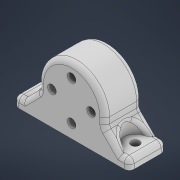
# Autodesk Inventor part: 15mm Hex Hub
Saved by Autodesk Inventor 2022 (Build 260153000, 153)
## iProperties
Created: 2021-11-10
Part Number: 15mm Hex Hub
Material: Generic
Document SubType Name: Modeling
Designer: izack
Density: 1 g/cm^3
Appearance: Default
Author: izack
## iProperties of the stored document 15mm Hex Hub_3DPrint.ipt
Part Number: 15mm Hex Hub_3DPrint
Material: Generic
Document SubType Name: Modeling
Designer: izack
Appearance: Default
Author: izack
Autodesk Inventor part; units mm, degrees
ref_plane "YZ Plane" through (0, 0, 0) normal (1, 0, 0) x (0, 1, 0)
ref_plane "XZ Plane" through (0, 0, 0) normal (0, 1, 0) x (-1, 0, 0)
ref_plane "XY Plane" through (0, 0, 0) normal (0, 0, 1) x (1, 0, 0)
sketch "Sketch1" plane through (0, 0, 0) normal (0, 0, 1) x (1, 0, 0)
  circle A0 centre (0, -10.5) radius 10.5 projected
  circle A1 centre (8, -10.5) radius 1.5 projected
  circle A2 centre (0, -2.5) radius 1.245 projected
  circle A3 centre (-8, -10.5) radius 1.5 projected
  circle A4 centre (0, -18.5) radius 1.245 projected
  circle A5 centre (0, -10.5) radius 13.5
  line L0 (0, -21) -> (13.5, -21)
  line L1 (23.5, -21) -> (23.5, -24)
  line L2 (0, -21) -> (-13.5, -21)
  line L3 (13.5, -10.5) -> (13.5, -21)
  line L4 (-13.5, -10.5) -> (-13.5, -21)
  circle A6 centre (8, -10.5) radius 1.75
  circle A7 centre (-8, -10.5) radius 1.75
  circle A8 centre (0, -2.5) radius 1.75
  circle A9 centre (0, -18.5) radius 1.75
  line L5 (13.5, -20) -> (23.5, -20)
  line L6 (23.5, -20) -> (23.5, -24)
  line L7 (23.5, -24) -> (-21.5, -24)
  line L8 (-23.5, -21) -> (-23.5, -20)
  line L9 (-23.5, -20) -> (-13.5, -20)
  line L10 (-23.5, -21) -> (-23.5, -24)
  line L11 (-23.5, -24) -> (-21.5, -24)
  point P0 (0, 0)
  point P1 (0, -24)
  dimension "d0" = 27
  dimension "d4" = 3.5
  dimension "d5" = 3.5
  dimension "d6" = 3.5
  dimension "d7" = 3.5
  dimension "d11" = 1
  dimension "d12" = 10
  dimension "d13" = 10
  constraints: 24 end point, 6 point on line, 5 centre point, 5 coincident, 4 point on circle, 4 tangent, 3 perpendicular, 2 horizontal, 1 collinear, 1 parallel, 1 vertical
  measures "d0" diameter of A5
  measures "d4" diameter of A6
  measures "d5" diameter of A7
  measures "d6" diameter of A8
  measures "d7" diameter of A9
  measures "d11" distance between parallel lines of L2 L9
  measures "d12" distance of L8.end L9.end
  measures "d13" distance of L5.start L5.end
extrude "Extrusion1" add sketch "Sketch1" along normal blind 15 contours A0 | L2 A5 L0 | L0 A5 L2 | L0 L3 L5 L6 L1 L7 A5 | A5 L3 L0 | L2 L4 A5 | A5 L7 L11 L10 L8 L9 L4 L2
sketch "Sketch2" plane through (13.5, -20, 0) normal (0, 1, 0) x (1, 0, 0)
  line L0 (-27, 0) -> (-37, 0) construction
  line L1 (-37, 0) -> (-27, 0) construction
  line L2 (-27, 0) -> (-32, 0) construction
  line L3 (-27, -15) -> (-37, -15) construction
  line L4 (-32, -15) -> (-32, 0) construction
  line L5 (10, 0) -> (0, 0) construction
  line L6 (5, 0) -> (5, -15) construction
  line L7 (10, -15) -> (0, -15) construction
  circle A0 centre (-32, -7.5) radius 1.7
  circle A1 centre (5, -7.5) radius 1.7
  circle A2 centre (-32, -7.5) radius 4.5
  circle A3 centre (5, -7.5) radius 4.5
  point P0 (-13.5, 0)
  dimension "d14" = 3.4
  dimension "d15" = 3.4
  dimension "d16" = 9
  dimension "d17" = 9
  constraints: 8 end point, 6 midpoint, 4 centre point, 2 coincident, 1 horizontal, 1 perpendicular
  measures "d14" diameter of A0
  measures "d15" diameter of A1
  measures "d16" diameter of A2
  measures "d17" diameter of A3
extrude "Extrusion2" cut sketch "Sketch2" against normal blind 15 contours A0 | A1
chamfer "Chamfer1" distance 6.25 angle 45 2 edges at (-13.5, -20, 7.5) (13.5, -20, 7.5)
extrude "Extrusion4" cut sketch "Sketch2" along normal blind 15
fillet "Fillet1" radius 2 25 edges at (23.5, -22, 15) (23.5, -22, 0) (-23.5, -22, 0) (-23.5, -22, 15) (-13.5, -12.125, 0) (13.5, -12.125, 0) (0, 3, 0) (-13.5, -12.125, 15) (13.5, -12.125, 15) (0, 3, 15) (16.625, -16.875, 15) (16.625, -16.875, 0) (-16.625, -16.875, 0) (-16.625, -16.875, 15) (21.625, -20, 0) (23.5, -20, 7.5) (21.625, -20, 15) (-21.625, -20, 0) (-23.5, -20, 7.5) (-21.625, -20, 15) (-15.7958, -16.0458, 3.9031) (-15.7958, -16.0458, 11.0969) (14, -14.25, 7.5) (13.5, -13.75, 7.5) (-13.5, -13.75, 7.5)
body "Solid1"
